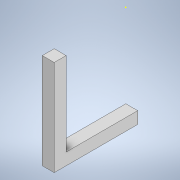
# Autodesk Inventor part: support
Saved by Autodesk Inventor 2020 (Build 240168000, 168)
## iProperties
Created: 2020-10-20
Part Number: support
Material: Generic
Document SubType Name: Modeling
Designer: maza168
Density: 1 g/cm^3
Appearance: Default
Author: maza168
Autodesk Inventor part; units mm, degrees
ref_plane "YZ Plane" through (0, 0, 0) normal (1, 0, 0) x (0, 1, 0)
ref_plane "XZ Plane" through (0, 0, 0) normal (0, 1, 0) x (-1, 0, 0)
ref_plane "XY Plane" through (0, 0, 0) normal (0, 0, 1) x (1, 0, 0)
sketch "Sketch1" plane through (0, 0, 0) normal (0, 0, 1) x (1, 0, 0)
  line L0 (0, 0) -> (20, 0)
  line L1 (20, 0) -> (20, 20)
  line L2 (20, 20) -> (0, 20)
  line L3 (0, 20) -> (0, 0)
  dimension "d0" = 20
  dimension "d1" = 20
  constraints: 8 end point, 2 parallel, 1 horizontal, 1 perpendicular
  measures "d0" distance of L0.start L0.end
  measures "d1" distance of L2.end L0.start
extrude "Extrusion1" add sketch "Sketch1" along normal blind 140
sketch "Sketch2" plane through (0, 20, 0) normal (0, 1, 0) x (1, 0, 0)
  line L0 (20, -140) -> (0, -140) projected
  line L1 (20, 0) -> (20, -140) projected
  line L2 (0, -140) -> (20, -140)
  line L3 (20, -140) -> (20, -120)
  line L4 (20, -120) -> (0, -120)
  line L5 (0, -120) -> (0, -140)
  point P0 (0, 0)
  dimension "d4" = 20
  constraints: 8 end point, 2 parallel, 1 horizontal, 1 perpendicular, 1 point on line
  measures "d4" distance of L4.end L0.end
extrude "Extrusion2" add sketch "Sketch2" along normal blind 140
sketch "Sketch3" plane through (0, 160, 0) normal (0, 1, 0) x (1, 0, 0)
  point P0 (0, 0)
body "Solid1"
